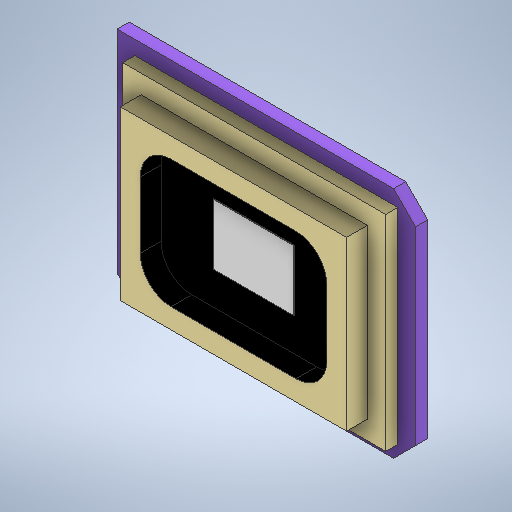
# Autodesk Inventor part: DLP
Saved by Autodesk Inventor 2025.1 (Build 291241000, 241)
## iProperties
Created: 2024-09-23
Part Number: DLP
Material: Generic
Document SubType Name: Modeling
Designer: PC
Density: 1 g/cm^3
Appearance: Default
Author: PC
Autodesk Inventor part; units mm, degrees
ref_plane "YZ Plane" through (0, 0, 0) normal (1, 0, 0) x (0, 1, 0)
ref_plane "XZ Plane" through (0, 0, 0) normal (0, 1, 0) x (-1, 0, 0)
ref_plane "XY Plane" through (0, 0, 0) normal (0, 0, 1) x (1, 0, 0)
sketch "Sketch1" plane through (0, 0, 0) normal (0, 0, 1) x (1, 0, 0)
  line L0 (3, 0) -> (40.64, 0)
  line L1 (37.65, 31.8) -> (0, 31.8)
  line L2 (0, 31.8) -> (0, 3)
  line L3 (37.65, 31.8) -> (40.65, 28.8)
  line L4 (3, 0) -> (0, 3)
  line L5 (40.65, 3) -> (37.65, 0)
  line L6 (40.65, 28.8) -> (40.65, 3)
  point P0 (0, 0)
  dimension "d4" = 3
  dimension "d5" = 45
  dimension "d6" = 45
  dimension "d7" = 3
  dimension "d8" = 31.8
  dimension "d9" = 40.65
  dimension "d10" = 3
  constraints: 14 end point, 10 coincident, 3 point on line, 1 horizontal, 1 parallel, 1 perpendicular, 1 vertical
  measures "d4" horizontal distance of L5.end L5.start
  measures "d5" angle of L0 L5
  measures "d6" angle of L1 L3
  measures "d7" horizontal distance of L0.start L2.end
  measures "d8" vertical distance of L0.start L1.end
  measures "d9" distance between parallel lines of L2 L6
  measures "d10" horizontal distance of L3.end L1.start
extrude "Extrusion1" add sketch "Sketch1" along normal blind 1.651
sketch "Sketch2" plane through (0, 0, 1.651) normal (0, 0, 1) x (1, 0, 0)
  line L0 (2.418, 29.87) -> (38.232, 29.87)
  line L1 (38.232, 29.87) -> (38.232, 1.93)
  line L2 (38.232, 1.93) -> (2.418, 1.93)
  line L3 (2.418, 1.93) -> (2.418, 29.87)
  line L4 (0, 31.8) -> (0, 3) projected
  line L5 (3, 0) -> (37.65, 0) projected
  line L6 (40.65, 3) -> (40.65, 28.8) projected
  point P0 (0, 0)
  point P1 (0, 17.4)
  point P2 (20.325, 1.93)
  point P3 (20.325, 0)
  point P4 (38.232, 15.9)
  point P5 (40.65, 15.9)
  dimension "d13" = 27.94
  dimension "d14" = 35.814
  constraints: 8 end point, 5 midpoint, 2 parallel, 1 horizontal, 1 horizontal alignment, 1 perpendicular, 1 vertical alignment
  measures "d13" distance of L2.end L0.start
  measures "d14" distance of L1.end L2.end
extrude "Extrusion2" add sketch "Sketch2" along normal blind 1.65
sketch "Sketch3" plane through (0, 0, 3.301) normal (0, 0, 1) x (1, 0, 0)
  line L0 (4.925, 27.33) -> (35.725, 27.33)
  line L1 (35.725, 27.33) -> (35.725, 4.47)
  line L2 (35.725, 4.47) -> (4.925, 4.47)
  line L3 (4.925, 4.47) -> (4.925, 27.33)
  line L4 (2.418, 29.87) -> (2.418, 1.93) projected
  line L5 (3, 0) -> (37.65, 0) projected
  point P0 (0, 0)
  point P1 (4.925, 15.9)
  point P2 (2.418, 15.9)
  point P3 (20.325, 4.47)
  point P4 (20.325, 0)
  dimension "d17" = 22.86
  dimension "d18" = 30.8
  constraints: 8 end point, 4 midpoint, 2 parallel, 1 horizontal, 1 horizontal alignment, 1 perpendicular, 1 vertical alignment
  measures "d17" distance between parallel lines of L2 L0
  measures "d18" distance of L1.end L2.end
extrude "Extrusion3" add sketch "Sketch3" along normal blind 2.83
sketch "Sketch4" plane through (0, 0, 6.131) normal (0, 0, 1) x (1, 0, 0)
  line L0 (11.825, 24.6) -> (28.825, 24.6)
  line L1 (33.025, 20.4) -> (33.025, 11.4)
  line L2 (28.825, 7.2) -> (11.825, 7.2)
  line L3 (7.625, 11.4) -> (7.625, 20.4)
  line L4 (4.925, 27.33) -> (4.925, 4.47) projected
  line L5 (2.418, 1.93) -> (38.232, 1.93) projected
  arc A0 (7.625, 11.4) -> (11.825, 7.2) centre (11.825, 11.4) ccw
  arc A1 (11.825, 24.6) -> (7.625, 20.4) centre (11.825, 20.4) ccw
  arc A2 (33.025, 20.4) -> (28.825, 24.6) centre (28.825, 20.4) ccw
  arc A3 (28.825, 7.2) -> (33.025, 11.4) centre (28.825, 11.4) ccw
  point P0 (0, 0)
  point P1 (7.625, 24.6)
  point P2 (33.025, 7.2)
  point P3 (7.625, 7.2)
  point P4 (7.625, 15.9)
  point P5 (4.925, 15.9)
  point P6 (20.325, 7.2)
  point P7 (20.325, 1.93)
  dimension "d21" = 17.4
  dimension "d22" = 25.4
  dimension "d23" = 4.2
  constraints: 8 end point, 8 point on circle, 8 tangent, 6 point on line, 4 centre point, 4 midpoint, 3 equal radius, 2 parallel, 1 horizontal, 1 horizontal alignment, 1 perpendicular, 1 vertical alignment
  measures "d21" distance of point (7.625, 7.2) point (7.625, 24.6)
  measures "d22" distance of point (33.025, 7.2) point (7.625, 7.2)
  measures "d23" radius of A0
extrude "Extrusion4" cut sketch "Sketch4" against normal blind 2.83
sketch "Sketch5" plane through (0, 0, 3.301) normal (0, 0, 1) x (1, 0, 0)
  line L0 (25.825, 11.775) -> (14.825, 11.775)
  line L1 (14.825, 11.775) -> (14.825, 20.025)
  line L2 (14.825, 20.025) -> (25.825, 20.025)
  line L3 (25.825, 20.025) -> (25.825, 11.775)
  line L4 (7.625, 11.4) -> (7.625, 20.4) projected
  line L5 (28.825, 7.2) -> (11.825, 7.2) projected
  point P0 (0, 0)
  point P1 (14.825, 15.9)
  point P2 (7.625, 15.9)
  point P3 (20.325, 11.775)
  point P4 (20.325, 7.2)
  dimension "d26" = 11
  dimension "d27" = 8.25
  constraints: 8 end point, 4 midpoint, 2 parallel, 1 horizontal, 1 horizontal alignment, 1 perpendicular, 1 vertical alignment
  measures "d26" distance between parallel lines of L1 L3
  measures "d27" distance of L0.end L1.end
extrude "Extrusion5" add sketch "Sketch5" along normal blind 0.1
body "Solid1"
